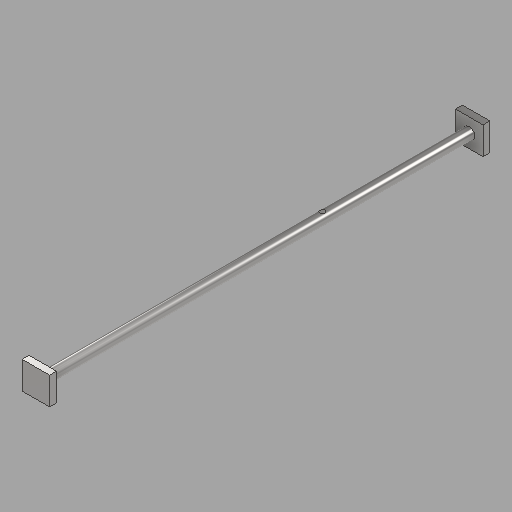
# Autodesk Inventor part: rear axle
Saved by Autodesk Inventor 2024 (Build 280153000, 153)
## iProperties
Created: 2024-04-12
Part Number: rear axle
Material: Steel, Mild
Document SubType Name: Modeling
Designer: Alex
Density: 7.85 g/cm^3
Appearance: Semi-Polished
Author: Alex
Autodesk Inventor part; units mm, degrees
ref_plane "YZ Plane" through (0, 0, 0) normal (1, 0, 0) x (0, 1, 0)
sketch "Sketch3" plane through (0, 0, 0) normal (0, 0, 1) x (1, 0, 0)
  circle A0 centre (0, 0) radius 4
  dimension "d11" = 8
  constraints: 1 centre point, 1 coincident
  measures "d11" diameter of A0
extrude "Extrusion5" add sketch "Sketch3" against normal blind 310
sketch "Sketch4" plane through (0, 0, 0) normal (0, 0, 1) x (1, 0, 0)
  line L0 (-10, 10) -> (10, 10)
  line L1 (10, 10) -> (10, -10)
  line L2 (10, -10) -> (-10, -10)
  line L3 (-10, -10) -> (-10, 10)
  line L4 (-10, 10) -> (10, -10) construction
  line L5 (10, 10) -> (-10, -10) construction
  point P0 (0, 0)
  dimension "d17" = 20
  dimension "d18" = 20
  constraints: 12 end point, 2 midpoint, 2 parallel, 1 horizontal, 1 perpendicular
  measures "d17" distance of L1.end L2.end
  measures "d18" distance of L0.end L1.end
extrude "Extrusion6" add sketch "Sketch4" along normal blind 5
ref_plane "Work Plane4" through (0, 0, -155) normal (0, 0, -1) x (-1, 0, 0)
mirror "Mirror1" about plane through (0, 0, -155) normal (0, 0, -1) of "Extrusion6"
ref_plane "Work Plane6" through (10, 10, -315) normal (0, -1, 0) x (-1, 0, 0)
ref_plane "Work Plane5" through (10, -10, -203.19) normal (0, 0, -1) x (-1, 0, 0)
sketch "Sketch5" plane through (10, 10, -315) normal (0, -1, 0) x (-1, 0, 0)
  line L0 (-4, -111.81) -> (24, -111.81) construction
  line L1 (14, -5) -> (6, -5) construction
  line L2 (6, -315) -> (14, -315) construction
  line L3 (0, -5) -> (20, -5) construction
  line L4 (10, -5) -> (10, -315) construction
  line L5 (6, -315) -> (6, -5) construction
  point P0 (10, -111.81)
  constraints: 2 end point, 2 midpoint, 1 parallel, 1 point on line
hole "Hole1" at (0, 10, -203.19) direction (0, -1, 0) diameter 3.688 end through all
body "Solid3"
